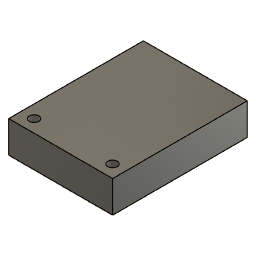
mouth_base_mount (Autodesk Fusion 360 design; units mm, degrees)
Autodesk Fusion 360 part; units mm, degrees
sketch "Sketch1" plane through (0, 0, 0) normal (0, 1, 0) x (1, 0, 0)
  line L0 (32.8, 42.5) -> (-32.8, 42.5)
  line L1 (-32.8, 42.5) -> (-32.8, -42.5)
  line L2 (-32.8, -42.5) -> (32.8, -42.5)
  line L3 (32.8, -42.5) -> (32.8, 42.5)
  line L4 (32.8, 42.5) -> (-32.8, -42.5) construction
  line L5 (-32.8, 42.5) -> (32.8, -42.5) construction
  dimension "d1" = 65.6
  dimension "d2" = 85
  constraint horizontal L0
  constraint perpendicular L0 L1
  constraint parallel L0 L2
  constraint parallel L1 L3
  constraint coincident L4 origin
  constraint coincident L5 origin
  measures "d1" distance of L1.end L2.end
  measures "d2" distance of L0.end L1.end
extrude "Extrude1" add sketch "Sketch1" along normal blind 20
sketch "Sketch2" plane through (0, 20, 0) normal (0, 1, 0) x (-1, 0, 0)
  line L0 (-32.8, 42.5) -> (-32.8, -42.5)
  line L1 (-32.8, -42.5) -> (32.8, -42.5)
  line L2 (32.8, -42.5) -> (32.8, 42.5)
  line L3 (32.8, 42.5) -> (-32.8, 42.5)
  line L4 (0, 42.5) -> (0, 34.5) construction
  line L5 (0, 34.5) -> (-24.75, 34.5) construction
  line L6 (0, 34.5) -> (24.75, 34.5) construction
  circle A0 centre (24.75, 34.5) radius 3
  circle A1 centre (-24.75, 34.5) radius 3
  dimension "d5" = 8
  dimension "d6" = 24.75
  dimension "d7" = 24.75
  dimension "d8" = 6
  dimension "d9" = 6
  constraint midpoint L3 L4.start
  constraint perpendicular L3 L4
  constraint perpendicular L4 L5
  constraint perpendicular L4 L6
  constraint coincident L6.end A0.centre
  constraint coincident L5.end A1.centre
  measures "d5" distance of L4.start L4.end
  measures "d6" distance of L4.end L5.end
  measures "d7" distance of L4.end L6.end
  measures "d8" diameter of A0
  measures "d9" diameter of A1
extrude "Extrude2" cut sketch "Sketch2" against normal up to surface (20 mm away) contours A0 | A1
ref_plane "WorkPlane1" through (0, 12, 0) normal (0, 1, 0) x (0, 0, 1)
sketch "Sketch3" plane through (0, 12, 0) normal (0, 1, 0) x (1, 0, 0)
  line L0 (20.0157, -34.5) -> (22.3829, -38.6)
  line L1 (22.3829, -38.6) -> (27.1171, -38.6)
  line L2 (27.1171, -38.6) -> (29.4843, -34.5)
  line L3 (29.4843, -34.5) -> (27.1171, -30.4)
  line L4 (27.1171, -30.4) -> (22.3829, -30.4)
  line L5 (22.3829, -30.4) -> (20.0157, -34.5)
  circle A0 centre (24.75, -34.5) radius 3
  line L6 (-20.0157, -34.5) -> (-22.3829, -30.4)
  line L7 (-22.3829, -30.4) -> (-27.1171, -30.4)
  line L8 (-27.1171, -30.4) -> (-29.4843, -34.5)
  line L9 (-29.4843, -34.5) -> (-27.1171, -38.6)
  line L10 (-27.1171, -38.6) -> (-22.3829, -38.6)
  line L11 (-22.3829, -38.6) -> (-20.0157, -34.5)
  circle A1 centre (-24.75, -34.5) radius 3
  point P0 (24.75, -34.5)
  point P1 (-24.75, -34.5)
  dimension "d13" = 4.1
  dimension "d14" = 4.1
  constraint coincident P0 A0.centre
  constraint coincident P1 A1.centre
  constraint horizontal L7
  constraint horizontal L4
  measures "d13" distance of P0 L5
  measures "d14" distance of P1 L11
extrude "Extrude3" cut sketch "Sketch3" against normal up to surface (12 mm away) contours L0 L1 L2 L3 L4 L5 | A0 | L6 L7 L8 L9 L10 L11 | A1
equation "d6 = ( 49.5 / 2 ) * 1 mm"
equation "d7 = ( 49.5 / 2 ) * 1 mm"
equation "d13 = ( 8.2 / 2 ) * 1 mm"
equation "d14 = ( 8.2 / 2 ) * 1 mm"
